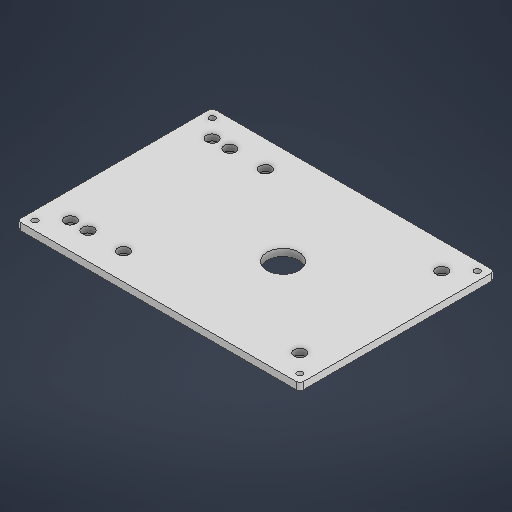
# Autodesk Inventor part: plate 2 for print
Saved by Autodesk Inventor 2025.2 (Build 292293000, 293)
## iProperties
Created: 2025-04-19
Part Number: plate 2 for print
Material: Generic
Document SubType Name: Modeling
Designer: klawy
Density: 1 g/cm^3
Appearance: Default
Author: klawy
Autodesk Inventor part; units mm, degrees
ref_plane "YZ Plane" through (0, 0, 0) normal (1, 0, 0) x (0, 1, 0)
ref_plane "XZ Plane" through (0, 0, 0) normal (0, 1, 0) x (-1, 0, 0)
ref_plane "XY Plane" through (0, 0, 0) normal (0, 0, 1) x (1, 0, 0)
sketch "Sketch1" plane through (0, 0, 0) normal (0, 1, 0) x (-1, 0, 0)
  line L0 (69.75, 45) -> (-69.75, 45)
  line L1 (-69.75, 45) -> (-69.75, -45)
  line L2 (-69.75, -45) -> (69.75, -45)
  line L3 (69.75, -45) -> (69.75, 45)
  line L4 (69.75, 45) -> (-69.75, -45) construction
  line L5 (-69.75, 45) -> (69.75, -45) construction
  circle A0 centre (-15.25, 0) radius 14.5
  line L6 (152.1746, 0) -> (-152.1746, 0) construction
  line L7 (0, 58.0523) -> (0, -58.0523) construction
  point P0 (0, 0)
  dimension "d0" = 139.5
  dimension "d2" = 29
  dimension "d4" = 90
  dimension "d5" = 54.5
  constraints: 16 end point, 4 midpoint, 2 horizontal, 2 parallel, 1 centre point, 1 perpendicular, 1 point on line, 1 vertical
  measures "d0" distance of L1.end L2.end
  measures "d2" diameter of A0
  measures "d4" distance of L0.end L1.end
  measures "d5" distance from line of L1 A0.centre
extrude "Extrusion1" add sketch "Sketch1" along normal blind 10
sketch "Sketch2" plane through (0, 10, 0) normal (0, 1, 0) x (1, 0, 0)
  line L0 (-64.75, -40) -> (64.75, -40) construction
  line L1 (64.75, -40) -> (64.75, 40) construction
  line L2 (64.75, 40) -> (-64.75, 40) construction
  line L3 (-64.75, 40) -> (-64.75, -40) construction
  line L4 (-64.75, -40) -> (64.75, 40) construction
  line L5 (64.75, -40) -> (-64.75, 40) construction
  line L6 (69.75, 45) -> (-69.75, 45) projected
  line L7 (69.75, -45) -> (69.75, 45) projected
  point P0 (0, 0)
  dimension "d11" = 5
  dimension "d12" = 5
  constraints: 12 end point, 4 coincident, 2 midpoint, 2 parallel, 1 horizontal, 1 perpendicular
  measures "d11" distance between parallel lines of L6 L2
  measures "d12" distance between parallel lines of L7 L1
hole "Hole1" at (-64.75, 10, -40) at (64.75, 10, -40) at (64.75, 10, 40) at (-64.75, 10, 40) direction (0, -1, 0) diameter 3.4 end through all counterbore diameter 6.5 counterbore depth 3.4 clearance for "Socket Head Cap Screw ISO 4762" size "M3" standard "ISO"
sketch "Sketch3" plane through (0, 0, 0) normal (0, -1, 0) x (1, 0, 0)
  circle A0 centre (-64.75, 40) radius 3.25 projected
  circle A1 centre (-64.75, 40) radius 4
  circle A2 centre (-64.75, 40) radius 1.7 projected
  circle A3 centre (64.75, 40) radius 1.7 projected
  circle A4 centre (64.75, -40) radius 1.7 projected
  circle A5 centre (-64.75, -40) radius 1.7 projected
  line L0 (69.75, 45) -> (69.75, -45) projected
  line L1 (-69.75, 45) -> (69.75, 45) projected
  line L2 (-69.75, -45) -> (-69.75, 45) projected
  line L3 (69.75, -45) -> (-69.75, -45) projected
  circle A6 centre (64.75, 40) radius 4
  circle A7 centre (-64.75, -40) radius 4
  circle A8 centre (64.75, -40) radius 4
  point P0 (0, 0)
  dimension "d22" = 129.5
  dimension "d25" = 80
  dimension "d28" = 8
  dimension "d63" = 90
  dimension "d64" = 139.5
  constraints: 4 centre point, 1 coincident, 1 horizontal, 1 vertical, 6 other
  measures "d22" distance of A1.centre A6.centre
  measures "d25" distance of A1.centre A7.centre
  measures "d28" diameter of A1
  measures "d63" distance of L2.start L1.start
  measures "d64" distance of L1.start L0.start
extrude "Extrusion2" cut sketch "Sketch3" against normal blind 1 contours A0 | A1 | A2 | A3 | A4 | A5 | A6 | A7 | A8
sketch "Sketch4" plane through (0, 0, 0) normal (0, -1, 0) x (1, 0, 0)
  circle A0 centre (64.75, -40) radius 4 projected
  circle A1 centre (-64.75, -40) radius 4 projected
  circle A2 centre (64.75, 40) radius 4 projected
  circle A3 centre (-64.75, 40) radius 4 projected
  line L0 (69.75, 45) -> (69.75, -45) projected
  line L1 (-69.75, 45) -> (69.75, 45) projected
  line L2 (-69.75, -45) -> (-69.75, 45) projected
  line L3 (69.75, -45) -> (-69.75, -45) projected
  circle A4 centre (15.25, 0) radius 14.5 projected
  circle A5 centre (15.25, 0) radius 17.5
  point P0 (0, 0)
  dimension "d31" = 35
  constraints: 1 centre point, 1 coincident
  measures "d31" diameter of A5
extrude "Extrusion3" cut sketch "Sketch4" against normal blind 5 contours A5
sketch "Sketch5" plane through (0, 0, 0) normal (0, -1, 0) x (1, 0, 0)
  line L0 (-59.75, 45) -> (-29.75, 45) construction
  line L1 (-29.75, 45) -> (-29.75, -45) construction
  line L2 (-29.75, -45) -> (-59.75, -45) construction
  line L3 (-59.75, -45) -> (-59.75, 45) construction
  line L4 (-97.65, 0) -> (97.65, 0) projected
  circle A0 centre (-54.75, 40) radius 4
  circle A1 centre (-34.75, 40) radius 4
  circle A2 centre (-54.75, -40) radius 4
  circle A3 centre (-34.75, -40) radius 4
  line L5 (-59.75, 45) -> (-29.75, -45) construction
  line L6 (-69.75, -45) -> (-69.75, 45) projected
  point P0 (0, 0)
  point P1 (-59.75, 0)
  point P2 (-44.75, 0)
  dimension "d34" = 90
  dimension "d35" = 30
  dimension "d36" = 8
  dimension "d37" = 5
  dimension "d38" = 5
  dimension "d41" = 20
  dimension "d44" = 80
  dimension "d47" = 25
  dimension "d65" = 90
  constraints: 10 end point, 4 centre point, 2 horizontal, 2 midpoint, 2 parallel, 1 perpendicular, 1 point on line, 1 vertical, 6 other
  measures "d34" distance of L2.end L0.start
  measures "d35" distance of L0.start L0.end
  measures "d36" diameter of A0
  measures "d37" distance from line of L0 A0.centre
  measures "d38" distance from line of L3 A0.centre
  measures "d41" distance of A0.centre A1.centre
  measures "d44" distance of A0.centre A2.centre
  measures "d47" distance from line of L6 point (-44.75, 0)
  measures "d65" distance of L6.start L6.end
extrude "Extrusion4" cut sketch "Sketch5" against normal blind 1
sketch "Sketch7" plane through (0, 10, 0) normal (0, 1, 0) x (1, 0, 0)
  circle A0 centre (-54.75, -40) radius 4 construction
  point P0 (0, 0)
  constraints: 1 coincident
hole "Hole2" at (-54.75, 10, 40) direction (0, -1, 0) diameter 3.4 end through all counterbore diameter 6.5 counterbore depth 3.4 clearance for "Socket Head Cap Screw ISO 4762" size "M3" standard "ISO"
pattern_linear "Rectangular Pattern1" count 2 spacing 80 along (0, 0, -1) count 2 spacing 20 along (1, 0, 0) of "Hole2"
sketch "Sketch8" plane through (0, 10, 0) normal (0, 1, 0) x (1, 0, 0)
  circle A0 centre (-34.75, 40) radius 3.25 projected
  circle A1 centre (-34.75, -40) radius 3.25 projected
  circle A2 centre (-54.75, 40) radius 3.25 projected
  circle A3 centre (-54.75, -40) radius 3.25 projected
  circle A4 centre (-64.75, -40) radius 3.25 projected
  circle A5 centre (64.75, -40) radius 3.25 projected
  circle A6 centre (64.75, 40) radius 3.25 projected
  circle A7 centre (-64.75, 40) radius 3.25 projected
  line L0 (69.75, -45) -> (69.75, 45) projected
  line L1 (69.75, 45) -> (-69.75, 45) projected
  line L2 (-69.75, 45) -> (-69.75, -45) projected
  line L3 (-69.75, -45) -> (69.75, -45) projected
  circle A8 centre (15.25, 0) radius 14.5 projected
  circle A9 centre (15.25, 0) radius 9
  point P0 (0, 0)
  dimension "d66" = 18
  constraints: 1 centre point, 1 coincident
  measures "d66" diameter of A9
extrude "Extrusion5" add sketch "Sketch8" against normal blind 4 contours A8
sketch "Sketch9" plane through (0, 10, 0) normal (0, 1, 0) x (1, 0, 0)
  circle A0 centre (15.25, 0) radius 9 projected
  circle A1 centre (-34.75, 40) radius 3.25 projected
  circle A2 centre (-34.75, -40) radius 3.25 projected
  circle A3 centre (-54.75, 40) radius 3.25 projected
  circle A4 centre (-54.75, -40) radius 3.25 projected
  circle A5 centre (-64.75, -40) radius 3.25 projected
  circle A6 centre (64.75, -40) radius 3.25 projected
  circle A7 centre (64.75, 40) radius 3.25 projected
  circle A8 centre (-64.75, 40) radius 3.25 projected
  line L0 (69.75, -45) -> (69.75, 45) projected
  line L1 (69.75, 45) -> (-69.75, 45) projected
  line L2 (-69.75, 45) -> (-69.75, -45) projected
  line L3 (-69.75, -45) -> (69.75, -45) projected
  line L4 (-79.75, 55) -> (79.75, 55)
  line L5 (79.75, 55) -> (79.75, -55)
  line L6 (79.75, -55) -> (-79.75, -55)
  line L7 (-79.75, -55) -> (-79.75, 55)
  point P0 (0, 0)
  dimension "d69" = 10
  dimension "d70" = 10
  dimension "d71" = 10
  dimension "d72" = 10
  constraints: 8 end point, 2 parallel, 1 horizontal, 1 perpendicular
  measures "d69" distance between parallel lines of L1 L4
  measures "d70" distance between parallel lines of L7 L2
  measures "d71" distance between parallel lines of L0 L5
  measures "d72" distance between parallel lines of L3 L6
extrude "Extrusion6" add sketch "Sketch9" against normal blind 4 contours L4 L5 L6 L7
fillet "Fillet1" radius 2 8 edges at (-79.75, 8, 55) (-69.75, 3, 45) (69.75, 3, 45) (79.75, 8, 55) (79.75, 8, -55) (69.75, 3, -45) (-69.75, 3, -45) (-79.75, 8, -55)
sketch "Sketch11" plane through (0, 10, 0) normal (0, 1, 0) x (1, 0, 0)
  line L0 (74.75, -50) -> (-74.75, -50) construction
  line L1 (-74.75, -50) -> (-74.75, 50) construction
  line L2 (-74.75, 50) -> (74.75, 50) construction
  line L3 (74.75, 50) -> (74.75, -50) construction
  line L4 (-79.75, 53) -> (-79.75, -53) construction
  line L5 (77.75, 55) -> (-77.75, 55) construction
  line L6 (-77.75, -55) -> (77.75, -55) construction
  line L7 (79.75, -53) -> (79.75, 53) construction
  point P0 (0, 0)
  dimension "d87" = 5
  dimension "d88" = 5
  dimension "d89" = 5
  dimension "d90" = 5
  constraints: 8 end point, 4 coincident, 2 parallel, 1 horizontal, 1 perpendicular
  measures "d87" distance between parallel lines of L4 L1
  measures "d88" distance between parallel lines of L5 L2
  measures "d89" distance between parallel lines of L6 L0
  measures "d90" distance between parallel lines of L7 L3
hole "Hole4" at (-74.75, 10, 50) at (-74.75, 10, -50) at (74.75, 10, -50) at (74.75, 10, 50) direction (0, -1, 0) diameter 3.4 end through all clearance for "Socket Head Cap Screw ISO 4762" size "M3" standard "ISO"
equation "\"d34\" = d65"
body "Solid1"
